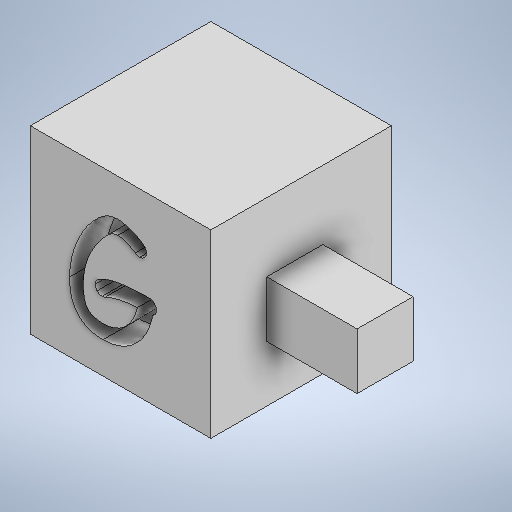
# Autodesk Inventor part: Guanine
Saved by Autodesk Inventor 2025 (Build 290162000, 162)
## iProperties
Created: 2024-08-12
Part Number: Guanine
Material: Generic
Document SubType Name: Modeling
Designer: kellst1
Density: 1 g/cm^3
Appearance: Default
Author: kellst1
Autodesk Inventor part; units mm, degrees
ref_plane "YZ Plane" through (0, 0, 0) normal (1, 0, 0) x (0, 1, 0)
ref_plane "XZ Plane" through (0, 0, 0) normal (0, 1, 0) x (-1, 0, 0)
ref_plane "XY Plane" through (0, 0, 0) normal (0, 0, 1) x (1, 0, 0)
sketch "Sketch1" plane through (0, 0, 0) normal (1, 0, 0) x (0, 1, 0)
  line L0 (0, 0) -> (10, 0)
  line L1 (10, 0) -> (10, -10)
  line L2 (10, -10) -> (0, -10)
  line L3 (0, -10) -> (0, 0)
  dimension "d0" = 10
  dimension "d1" = 10
  constraints: 8 end point, 2 parallel, 1 horizontal, 1 perpendicular
  measures "d0" distance of L1.end L2.end
  measures "d1" distance of L0.end L1.end
extrude "Extrusion1" add sketch "Sketch1" along normal blind 10
sketch "Sketch4" plane through (0, 0, 0) normal (0, 0, 1) x (1, 0, 0)
  line L0 (1.8731, 7.9408) -> (4.4271, 7.9408) construction
  line L1 (4.4271, 7.9408) -> (4.4271, 4.8928) construction
  line L2 (4.4271, 4.8928) -> (1.8731, 4.8928) construction
  line L3 (1.8731, 4.8928) -> (1.8731, 7.9408) construction
  spline S0 degree 2 poles (6.7794, 4.2913) (6.548, 3.1344) (5.0493, 1.7514) (4.0292, 1.7514) knots 0 0 0 1 2 2 2
  spline S1 degree 2 poles (4.0292, 1.7514) (3.0984, 1.7514) (2.1729, 2.7873) (2.1729, 3.8285) knots 0 0 0 1 2 2 2
  spline S2 degree 2 poles (2.1729, 3.8285) (2.1729, 4.8066) (3.0984, 6.8785) (3.8241, 7.5148) knots 0 0 0 1 2 2 2
  spline S3 degree 2 poles (3.8241, 7.5148) (4.3079, 7.9408) (4.8442, 7.9408) knots 0 0 0 1 1 1
  spline S4 degree 2 poles (4.8442, 7.9408) (5.1861, 7.9408) (5.7487, 7.7146) knots 0 0 0 1 1 1
  spline S5 degree 2 poles (5.7487, 7.7146) (6.4376, 7.4412) (6.4376, 7.1152) knots 0 0 0 1 1 1
  spline S6 degree 2 poles (6.4376, 7.1152) (6.4376, 6.9574) (6.2115, 6.7155) (6.0537, 6.7155) knots 0 0 0 1 2 2 2
  spline S7 degree 2 poles (6.0537, 6.7155) (5.9696, 6.7155) (5.8171, 6.8102) knots 0 0 0 1 1 1
  spline S8 degree 2 poles (5.8171, 6.8102) (5.2439, 7.1625) (4.8442, 7.1625) knots 0 0 0 1 1 1
  spline S9 degree 2 poles (4.8442, 7.1625) (4.5603, 7.1625) (4.25, 6.868) knots 0 0 0 1 1 1
  spline S10 degree 2 poles (4.25, 6.868) (4.0975, 6.7208) (3.8083, 6.3316) knots 0 0 0 1 1 1
  spline S11 degree 2 poles (3.8083, 6.3316) (2.9354, 5.18) (2.9354, 3.8285) knots 0 0 0 1 1 1
  spline S12 degree 2 poles (2.9354, 3.8285) (2.9354, 3.1186) (3.1562, 2.8346) knots 0 0 0 1 1 1
  spline S13 degree 2 poles (3.1562, 2.8346) (3.3929, 2.5244) (4.0292, 2.5244) knots 0 0 0 1 1 1
  spline S14 degree 2 poles (4.0292, 2.5244) (4.7023, 2.5244) (5.2018, 2.9503) knots 0 0 0 1 1 1
  spline S15 degree 2 poles (5.2018, 2.9503) (5.7277, 3.4026) (5.9328, 4.2439) knots 0 0 0 1 1 1
  spline S16 degree 2 poles (5.9328, 4.2439) (4.8916, 4.1914) (4.1448, 3.8443) knots 0 0 0 1 1 1
  spline S17 degree 2 poles (4.1448, 3.8443) (4.0554, 3.8022) (3.9766, 3.8022) knots 0 0 0 1 1 1
  spline S18 degree 2 poles (3.9766, 3.8022) (3.8083, 3.8022) (3.6979, 3.9284) knots 0 0 0 1 1 1
  spline S19 degree 2 poles (3.6979, 3.9284) (3.5979, 4.0494) (3.5979, 4.2019) knots 0 0 0 1 1 1
  spline S20 degree 2 poles (3.5979, 4.2019) (3.5979, 4.407) (3.7978, 4.5332) knots 0 0 0 1 1 1
  spline S21 degree 2 poles (3.7978, 4.5332) (4.6129, 5.0275) (6.6059, 5.0275) knots 0 0 0 1 1 1
  spline S22 degree 2 poles (6.6059, 5.0275) (6.7636, 5.0275) (6.9845, 4.8066) (6.9845, 4.6436) knots 0 0 0 1 2 2 2
  spline S23 degree 2 poles (6.9845, 4.6436) (6.9845, 4.3964) (6.7794, 4.2913) knots 0 0 0 1 1 1
  point P0 (0, 0)
  constraints: 2 other
extrude "Extrusion4" cut sketch "Sketch4" against normal blind 2
sketch "Sketch5" plane through (10, 0, 0) normal (1, 0, 0) x (0, 0, -1)
  line L0 (3.1, 3.1) -> (6.2, 3.1)
  line L1 (6.2, 3.1) -> (6.2, 6.2)
  line L2 (6.2, 6.2) -> (3.1, 6.2)
  line L3 (3.1, 6.2) -> (3.1, 3.1)
  point P0 (0, 0)
  dimension "d11" = 3.1
  dimension "d12" = 3.1
  constraints: 8 end point, 2 parallel, 1 horizontal, 1 perpendicular
  measures "d11" distance of L2.end L1.end
  measures "d12" distance of L1.end L0.end
extrude "Extrusion5" add sketch "Sketch5" along normal blind 5
body "Solid1"
